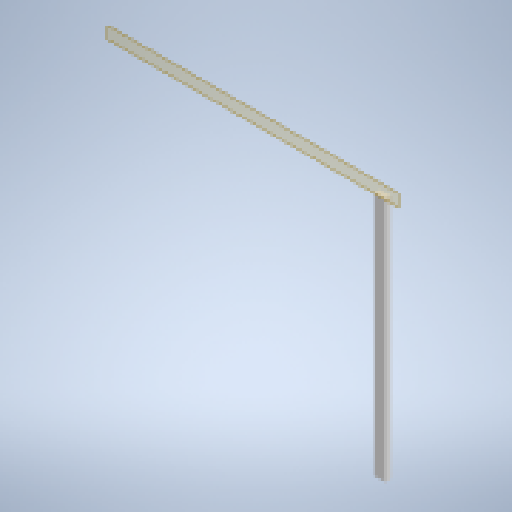
# Autodesk Inventor part: 7'5''x2x4
Saved by Autodesk Inventor 2025 (Build 290162000, 162)
## iProperties
Created: 2024-09-18
Part Number: 7'5''x2x4
Material: Generic
Document SubType Name: Modeling
Designer: localadmin
Density: 1 g/cm^3
Appearance: Default
Author: localadmin
Autodesk Inventor part; units mm, degrees
ref_plane "YZ Plane" through (0, 0, 0) normal (1, 0, 0) x (0, 1, 0)
ref_plane "XZ Plane" through (0, 0, 0) normal (0, 1, 0) x (-1, 0, 0)
ref_plane "XY Plane" through (0, 0, 0) normal (0, 0, 1) x (1, 0, 0)
ref_plane "Work Plane1" through (0, 0, 0) normal (0, 0, 1) x (1, 0, 0)
sketch "Sketch1" plane through (0, 0, 0) normal (0, 0, 1) x (1, 0, 0)
  line L0 (-1219.2, -2311.4) -> (-1219.2, -2413) projected
  line L1 (-1219.2, -2413) -> (1219.2, -2413) projected
  line L2 (1219.2, -2413) -> (1219.2, -2311.4) projected
  line L3 (1219.2, -2311.4) -> (-1219.2, -2311.4) projected
  line L4 (-1219.2, 50.8) -> (-1219.2, -50.8) projected
  line L5 (-1219.2, -50.8) -> (1219.2, -50.8) projected
  line L6 (1219.2, -50.8) -> (1219.2, 50.8) projected
  line L7 (1219.2, 50.8) -> (-1219.2, 50.8) projected
  line L8 (1219.2, -50.8) -> (1219.2, -2311.4)
  line L9 (1219.2, -2311.4) -> (1117.6, -2311.4)
  line L10 (1117.6, -2311.4) -> (1117.6, -50.8)
  line L11 (1117.6, -50.8) -> (1219.2, -50.8)
  point P0 (0, 0)
  dimension "d0" = 101.6
  constraints: 8 end point, 2 point on line, 1 collinear, 1 perpendicular, 1 vertical
  measures "d0" distance of L2.end L9.end
extrude "Extrusion1" add sketch "Sketch1" against normal blind 50.8 contours L10 L5 L8 L3
body "Solid1"
